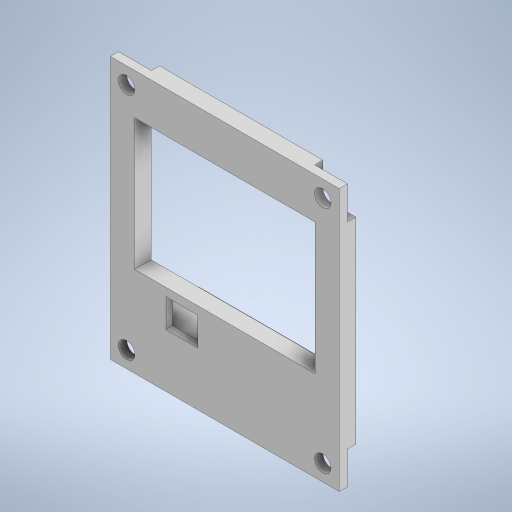
# Autodesk Inventor part: FrontPLate
Saved by Autodesk Inventor 2023 (Build 270158000, 158)
## iProperties
Created: 2023-09-26
Part Number: FrontPLate
Material: Generic
Document SubType Name: Modeling
Designer: Gage
Density: 1 g/cm^3
Appearance: Default
Author: Gage
## iProperties of the stored document FrontPLate_3DPrint.ipt
Created: 2023-10-27
Part Number: FrontPLate_3DPrint
Material: Generic
Document SubType Name: Modeling
Designer: Gage
Density: 1 g/cm^3
Appearance: Default
Author: Gage
Autodesk Inventor part; units mm, degrees
ref_plane "YZ Plane" through (0, 0, 0) normal (1, 0, 0) x (0, 1, 0)
ref_plane "XZ Plane" through (0, 0, 0) normal (0, 1, 0) x (-1, 0, 0)
ref_plane "XY Plane" through (0, 0, 0) normal (0, 0, 1) x (1, 0, 0)
sketch "Sketch1" plane through (0, 0, 0) normal (0, 0, 1) x (1, 0, 0)
  line L0 (-44.323, 50.8) -> (44.323, 50.8)
  line L1 (44.323, 50.8) -> (44.323, -50.8)
  line L2 (44.323, -50.8) -> (-44.323, -50.8)
  line L3 (-44.323, -50.8) -> (-44.323, 50.8)
  point P0 (0, 0)
  point P1 (0, 50.8)
  point P2 (44.323, 0)
  dimension "d0" = 88.646
  dimension "d1" = 101.6
  constraints: 8 end point, 2 midpoint, 2 parallel, 1 horizontal, 1 horizontal alignment, 1 perpendicular, 1 vertical alignment
  measures "d0" distance of L1.end L2.end
  measures "d1" distance of L0.end L1.end
extrude "Extrusion1" add sketch "Sketch1" along normal blind 6.35
sketch "Sketch2" plane through (0, 0, 0) normal (0, 0, -1) x (-1, 0, 0)
  line L0 (-44.323, 50.8) -> (44.323, 50.8) projected
  line L1 (-44.323, 50.8) -> (-31.623, 50.8)
  line L2 (-31.623, 50.8) -> (-31.623, 38.1)
  line L3 (-31.623, 38.1) -> (-44.323, 38.1)
  line L4 (-44.323, 38.1) -> (-44.323, 50.8)
  line L5 (44.323, 50.8) -> (31.623, 50.8)
  line L6 (31.623, 50.8) -> (31.623, 38.1)
  line L7 (31.623, 38.1) -> (44.323, 38.1)
  line L8 (44.323, 38.1) -> (44.323, 50.8)
  line L9 (44.323, -50.8) -> (-44.323, -50.8) projected
  line L10 (44.323, -50.8) -> (31.623, -50.8)
  line L11 (31.623, -50.8) -> (31.623, -38.1)
  line L12 (31.623, -38.1) -> (44.323, -38.1)
  line L13 (44.323, -38.1) -> (44.323, -50.8)
  line L14 (-44.323, -50.8) -> (-31.623, -50.8)
  line L15 (-31.623, -50.8) -> (-31.623, -38.1)
  line L16 (-31.623, -38.1) -> (-44.323, -38.1)
  line L17 (-44.323, -38.1) -> (-44.323, -50.8)
  point P0 (0, 0)
  dimension "d4" = 12.7
  dimension "d5" = 12.7
  dimension "d6" = 12.7
  dimension "d7" = 12.7
  dimension "d8" = 12.7
  dimension "d9" = 12.7
  dimension "d10" = 12.7
  dimension "d11" = 12.7
  constraints: 32 end point, 8 parallel, 4 horizontal, 4 perpendicular
  measures "d4" distance of L2.end L3.end
  measures "d5" distance of L1.end L2.end
  measures "d6" distance of L7.end L6.end
  measures "d7" distance of L6.end L5.end
  measures "d8" distance of L11.end L12.end
  measures "d9" distance of L10.end L11.end
  measures "d10" distance of L16.end L15.end
  measures "d11" distance of L15.end L14.end
extrude "Extrusion2" cut sketch "Sketch2" against normal blind 3.175
sketch "Sketch3" plane through (0, 0, 3.175) normal (0, 0, -1) x (-1, 0, 0)
  circle A0 centre (-37.973, 44.45) radius 3.175
  circle A1 centre (37.973, 44.45) radius 3.175
  circle A2 centre (37.973, -44.45) radius 3.175
  circle A3 centre (-37.973, -44.45) radius 3.175
  line L0 (-44.323, 50.8) -> (-31.623, 50.8) projected
  line L1 (-44.323, 38.1) -> (-44.323, 50.8) projected
  line L2 (31.623, 50.8) -> (44.323, 50.8) projected
  line L3 (44.323, 50.8) -> (44.323, 38.1) projected
  line L4 (44.323, -38.1) -> (44.323, -50.8) projected
  line L5 (44.323, -50.8) -> (31.623, -50.8) projected
  line L6 (-31.623, -50.8) -> (-44.323, -50.8) projected
  line L7 (-44.323, -50.8) -> (-44.323, -38.1) projected
  point P0 (0, 0)
  point P1 (-37.973, 50.8)
  point P2 (37.973, 50.8)
  point P3 (37.973, -50.8)
  point P4 (-37.973, -50.8)
  dimension "d14" = 6.35
  dimension "d15" = 6.35
  dimension "d16" = 6.35
  dimension "d17" = 6.35
  dimension "d18" = 6.35
  dimension "d19" = 6.35
  dimension "d20" = 6.35
  dimension "d21" = 6.35
  dimension "d22" = 6.35
  dimension "d23" = 6.35
  dimension "d24" = 6.35
  dimension "d25" = 6.35
  constraints: 4 centre point, 4 midpoint
  measures "d14" diameter of A0
  measures "d15" diameter of A1
  measures "d16" diameter of A2
  measures "d17" diameter of A3
  measures "d18" distance of point (-37.973, 50.8) A0.centre
  measures "d19" distance from line of L1 A0.centre
  measures "d20" distance of point (37.973, 50.8) A1.centre
  measures "d21" distance from line of L3 A1.centre
  measures "d22" distance from line of L4 A2.centre
  measures "d23" distance of point (37.973, -50.8) A2.centre
  measures "d24" distance of point (-37.973, -50.8) A3.centre
  measures "d25" distance from line of L7 A3.centre
extrude "Extrusion3" cut sketch "Sketch3" against normal blind 3.175
sketch "Sketch4" plane through (0, 0, 0) normal (0, 0, -1) x (-1, 0, 0)
  line L0 (-34.925, 34.925) -> (34.925, 34.925)
  line L1 (34.925, 34.925) -> (34.925, -15.875)
  line L2 (34.925, -15.875) -> (-34.925, -15.875)
  line L3 (-34.925, -15.875) -> (-34.925, 34.925)
  line L4 (-31.623, 50.8) -> (31.623, 50.8) projected
  point P0 (0, 0)
  point P1 (34.925, 9.525)
  point P2 (0, 34.925)
  dimension "d28" = 69.85
  dimension "d29" = 50.8
  dimension "d47" = 15.875
  constraints: 8 end point, 2 midpoint
  measures "d28" distance of L1.end L2.end
  measures "d29" distance of L0.end L1.end
  measures "d47" distance between parallel lines of L0 L4
extrude "Extrusion4" cut sketch "Sketch4" against normal blind 25.4
sketch "Sketch5" plane through (0, 0, 0) normal (0, 0, -1) x (-1, 0, 0)
  line L0 (-34.925, 34.925) -> (34.925, 34.925) projected
  line L1 (34.925, 34.925) -> (43.053, 34.925)
  line L2 (43.053, 34.925) -> (43.053, -15.875)
  line L3 (43.053, -15.875) -> (34.925, -15.875)
  line L4 (34.925, -15.875) -> (34.925, 34.925)
  line L5 (44.323, 50.8) -> (44.323, -50.8) projected
  line L6 (43.053, -15.875) -> (44.323, -15.875)
  line L7 (44.323, -15.875) -> (44.323, 34.925)
  line L8 (44.323, 34.925) -> (43.053, 34.925)
  line L9 (43.053, 34.925) -> (43.053, -15.875)
  line L10 (44.323, -15.875) -> (34.925, -15.875)
  line L11 (34.925, -15.875) -> (34.925, -17.4625)
  line L12 (34.925, -17.4625) -> (44.323, -17.4625)
  line L13 (44.323, -17.4625) -> (44.323, -15.875)
  point P0 (0, 0)
  point P1 (34.925, -15.875)
  point P2 (43.053, 34.925)
  dimension "d32" = 8.128
  dimension "d33" = 50.8
  dimension "d34" = 50.8
  constraints: 24 end point, 6 parallel, 3 horizontal, 3 perpendicular, 1 point on line
  measures "d32" distance of L2.end L3.end
  measures "d33" distance of L3.end L0.end
  measures "d34" distance of L7.end L6.end
extrude "Extrusion5" [suppressed]
sketch "Sketch6" plane through (-43.053, -15.875, 0) normal (0, 1, 0) x (1, 0, 0)
  line L0 (0, 3.6195) -> (8.128, 3.6195) projected
  line L1 (8.128, 0) -> (8.128, 3.6195) projected
  line L2 (0, 3.6195) -> (8.128, 3.6195)
  line L3 (8.128, 3.6195) -> (8.128, 2.032)
  line L4 (8.128, 2.032) -> (0, 2.032)
  line L5 (0, 2.032) -> (0, 3.6195)
  point P0 (43.053, 0)
  dimension "d37" = 1.5875
  constraints: 8 end point, 2 parallel, 1 horizontal, 1 perpendicular, 1 point on line
  measures "d37" distance of L2.end L3.end
extrude "Extrusion6" [suppressed]
sketch "Sketch7" plane through (0, 0, 0) normal (0, 0, -1) x (-1, 0, 0)
  line L0 (34.925, -15.875) -> (-34.925, -15.875) projected
  line L1 (-34.925, -15.875) -> (34.925, -15.875)
  line L2 (34.925, -15.875) -> (34.925, -17.4625)
  line L3 (34.925, -17.4625) -> (-34.925, -17.4625)
  line L4 (-34.925, -17.4625) -> (-34.925, -15.875)
  point P0 (0, 0)
  point P1 (34.925, -15.875)
  constraints: 8 end point, 2 parallel, 1 horizontal, 1 perpendicular
extrude "Extrusion7" [suppressed]
sketch "Sketch8" plane through (0, 0, 0) normal (0, 0, -1) x (-1, 0, 0)
  line L0 (10.4299, -18.9992) -> (22.7489, -18.9992)
  line L1 (22.7489, -18.9992) -> (22.7489, -29.9466)
  line L2 (22.7489, -29.9466) -> (10.4299, -29.9466)
  line L3 (10.4299, -29.9466) -> (10.4299, -18.9992)
  line L4 (31.623, -50.8) -> (-31.623, -50.8) projected
  line L5 (-44.323, -50.8) -> (-44.323, 50.8) projected
  line L6 (44.323, 38.1) -> (44.323, -38.1) projected
  point P0 (0, 0)
  point P1 (44.323, -17.4625)
  dimension "d42" = 12.319
  dimension "d43" = 10.9474
  dimension "d44" = 20.8534
  dimension "d51" = 21.5741
  constraints: 8 end point, 2 parallel, 1 horizontal, 1 perpendicular
  measures "d42" distance of L1.end L2.end
  measures "d43" distance of L0.end L1.end
  measures "d44" distance between parallel lines of L4 L2
  measures "d51" distance between parallel lines of L6 L1
extrude "Extrusion8" cut sketch "Sketch8" against normal through all
sketch "Sketch9" plane through (0, 0, 0) normal (0, 0, -1) x (-1, 0, 0)
  line L0 (10.4299, -18.9992) -> (22.7489, -18.9992) projected
  line L1 (10.4299, -18.9992) -> (-22.225, -18.9992)
  line L2 (-22.225, -18.9992) -> (-22.225, -29.9466)
  line L3 (-22.225, -29.9466) -> (10.4299, -29.9466)
  line L4 (10.4299, -29.9466) -> (10.4299, -18.9992)
  point P0 (0, 0)
  dimension "d55" = 10.9474
  constraints: 8 end point, 2 parallel, 1 horizontal, 1 perpendicular
  measures "d55" distance of L1.end L2.end
extrude "Extrusion9" cut sketch "Sketch9" against normal blind 3.175
shell "Shell1" thickness 2.54 removed faces 1 at (7.4083, -43.8489, 0)
sketch "Sketch10" plane through (0, 0, 0) normal (0, 0, -1) x (-1, 0, 0)
  line L0 (22.7489, -18.9992) -> (22.7489, -29.9466) projected
  line L1 (25.2889, -32.4866) -> (25.2889, -18.415) projected
  line L2 (22.7489, -18.9992) -> (25.2889, -18.9992)
  line L3 (25.2889, -18.9992) -> (25.2889, -32.4866)
  line L4 (25.2889, -32.4866) -> (22.7489, -32.4866)
  line L5 (22.7489, -32.4866) -> (22.7489, -18.9992)
  line L6 (-24.765, -32.4866) -> (-24.765, -18.415) projected
  line L7 (22.7489, -32.4866) -> (-24.765, -32.4866)
  line L8 (-24.765, -32.4866) -> (-24.765, -29.8771)
  line L9 (-24.765, -29.8771) -> (22.7489, -29.8771)
  line L10 (22.7489, -29.8771) -> (22.7489, -32.4866)
  line L11 (-22.225, -29.9466) -> (-22.225, -18.9992) projected
  line L12 (-24.765, -29.8771) -> (-22.225, -29.8771)
  line L13 (-22.225, -29.8771) -> (-22.225, -18.9992)
  line L14 (-22.225, -18.9992) -> (-24.765, -18.9992)
  line L15 (-24.765, -18.9992) -> (-24.765, -29.8771)
  point P0 (0, 0)
  point P1 (-22.225, -29.8771)
  constraints: 24 end point, 6 parallel, 3 horizontal, 3 perpendicular, 1 point on line
extrude "Extrusion10" cut sketch "Sketch10" against normal blind 3.81
sketch "Sketch12" plane through (0, 0, 3.175) normal (0, 0, -1) x (-1, 0, 0)
  line L0 (-22.225, -29.8771) -> (10.4299, -29.8771) projected
  line L1 (-22.225, -19.05) -> (10.4299, -19.05)
  line L2 (10.4299, -19.05) -> (10.4299, -29.8771)
  line L3 (10.4299, -29.8771) -> (-22.225, -29.8771)
  line L4 (-22.225, -29.8771) -> (-22.225, -19.05)
  line L5 (-22.225, -18.9992) -> (10.4299, -18.9992) projected
  line L6 (-22.225, -18.9992) -> (10.4299, -18.9992)
  line L7 (10.4299, -18.9992) -> (10.4299, -19.05)
  line L8 (10.4299, -19.05) -> (-22.225, -19.05)
  line L9 (-22.225, -19.05) -> (-22.225, -18.9992)
  point P0 (0, 0)
  constraints: 16 end point, 4 parallel, 2 horizontal, 2 perpendicular
extrude "Extrusion12" cut sketch "Sketch12" against normal blind 0.635
sketch "Sketch11" plane through (29.083, -48.26, 3.81) normal (0, 0, -1) x (-1, 0, 0)
  line L0 (4.8419, 14.7415) -> (63.2619, 14.7415)
  line L1 (63.2619, 14.7415) -> (63.2619, 12.2015)
  line L2 (63.2619, 12.2015) -> (4.8419, 12.2015)
  line L3 (4.8419, 12.2015) -> (4.8419, 14.7415)
  line L4 (39.5129, 18.3134) -> (51.8319, 18.3134) projected
  line L5 (51.8319, 18.3134) -> (51.8319, 29.2608) projected
  point P0 (29.083, 48.26)
  dimension "d58" = 3.5719
  dimension "d59" = 2.54
  dimension "d60" = 11.43
  dimension "d61" = 58.42
  constraints: 8 end point, 2 parallel, 1 horizontal, 1 perpendicular
  measures "d58" distance between parallel lines of L0 L4
  measures "d59" distance of L2.end L0.start
  measures "d60" distance between parallel lines of L1 L5
  measures "d61" distance of L1.end L2.end
extrude "Extrusion11" add sketch "Sketch11" along normal blind 21.59
sketch "Sketch13" plane through (-34.1789, -33.5185, 3.81) normal (0, 1, 0) x (1, 0, 0)
  circle A0 centre (5.08, 18.415) radius 1.5875
  line L0 (58.42, 0) -> (0, 0) projected
  circle A1 centre (53.34, 17.145) radius 1.5875
  line L1 (58.42, 0) -> (58.42, 21.59) projected
  line L2 (0, 0) -> (0, 21.59) projected
  circle A2 centre (5.08, 15.24) radius 1.5875
  circle A3 centre (53.34, 13.97) radius 1.5875
  line L3 (6.6675, 18.415) -> (6.6675, 15.24)
  line L4 (3.4925, 18.415) -> (3.4925, 15.24)
  line L5 (51.7525, 17.145) -> (51.7525, 13.97)
  line L6 (54.9275, 17.145) -> (54.9275, 13.6525)
  point P0 (34.1789, 3.81)
  point P1 (54.9275, 13.97)
  dimension "d84" = 3.175
  dimension "d66" = 3.175
  dimension "d67" = 18.415
  dimension "d68" = 3.175
  dimension "d69" = 17.145
  dimension "d70" = 5.08
  dimension "d71" = 5.08
  dimension "d83" = 3.175
  dimension "d85" = 3.175
  dimension "d86" = 3.175
  constraints: 8 end point, 6 point on circle, 3 centre point, 3 tangent, 2 parallel, 1 vertical, 3 other
  measures "d66" diameter of A0
  measures "d67" distance from line of A0.centre L0
  measures "d68" diameter of A1
  measures "d69" distance from line of L0 A1.centre
  measures "d70" distance from line of L1 A1.centre
  measures "d71" distance from line of L2 A0.centre
  measures "d83" diameter of A2
  measures "d85" distance of A2.centre A0.centre
  measures "d86" distance of A1.centre point (53.34, 13.97)
extrude "Extrusion13" cut sketch "Sketch13" against normal blind 31.75
sketch "Sketch16" plane through (0, 0, 0) normal (0, 0, -1) x (-1, 0, 0)
  line L0 (-37.465, -18.415) -> (-24.765, -18.415) projected
  line L1 (-22.225, -18.9992) -> (22.7489, -18.9992) projected
  line L2 (-24.765, -18.415) -> (25.2889, -18.415)
  line L3 (25.2889, -18.415) -> (25.2889, -18.9992)
  line L4 (25.2889, -18.9992) -> (-24.765, -18.9992)
  line L5 (-24.765, -18.9992) -> (-24.765, -18.415)
  point P0 (0, 0)
  point P1 (-24.765, -18.9992)
  point P2 (-24.765, -18.9992)
  point P3 (22.7489, -18.9992)
  constraints: 8 end point, 2 parallel, 1 horizontal, 1 perpendicular
extrude "Extrusion14" cut sketch "Sketch16" against normal blind 3.81
body "Solid1"
